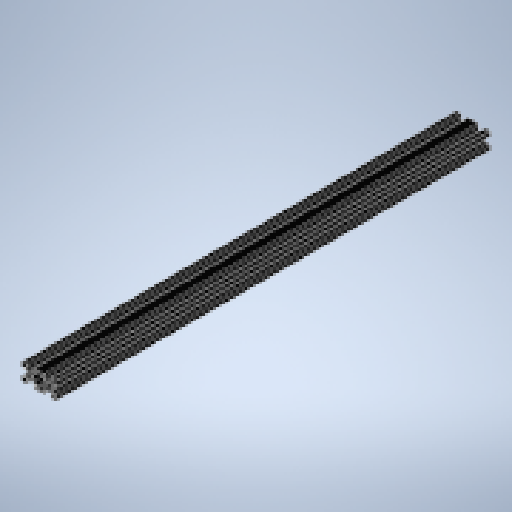
# Autodesk Inventor part: V-Slot_20x40_500
Saved by Autodesk Inventor 2025.1 (Build 291241020, 241B)
## iProperties
Created: 2017-01-26
Part Number: V-Slot_20x40_500
Material: Aluminum 6061
Document SubType Name: Modeling
Designer: leon-
Density: 2.7 g/cm^3
Appearance: Anodized - Black
Sending System: SolidWorks 2019
Last Author: ricardo
Last Saved: 2020-01-30
Author: leon-
Autodesk Inventor part; units mm, degrees
ref_plane "YZ Plane" through (0, 0, 0) normal (1, 0, 0) x (0, 1, 0)
ref_plane "XZ Plane" through (0, 0, 0) normal (0, 1, 0) x (-1, 0, 0)
ref_plane "Work Plane2" through (-5.2, 10, 100) normal (0, 0, 1) x (1, 0, 0)
sketch "Sketch1" plane through (-5.2, 10, 100) normal (0, 0, 1) x (1, 0, 0)
  line L0 (7.9, -18.2) -> (7.9, -16.2393) projected
  line L1 (2.5, -18.2) -> (7.9, -18.2) projected
  line L2 (2.5, -18.2) -> (2.5, -16.2393) projected
  line L3 (2.5, -16.2393) -> (-0.8, -12.9393) projected
  line L4 (-0.8, -7.0607) -> (-0.8, -12.9393) projected
  line L5 (2.5, -3.7607) -> (-0.8, -7.0607) projected
  line L6 (12.2, -18.2) -> (9.7, -18.2) projected
  line L7 (10.4, -20) -> (12.2, -18.2) projected
  line L8 (0, -20) -> (10.4, -20) projected
  line L9 (0, -20) -> (-1.8, -18.2) projected
  line L10 (-1.8, -18.2) -> (0.7, -18.2) projected
  line L11 (0.7, -18.2) -> (0.7, -16.5607) projected
  line L12 (0.7, -16.5607) -> (-1.8607, -14) projected
  line L13 (-1.8607, -14) -> (-4.5, -14) projected
  line L14 (-4.5, -14) -> (-4.8, -13.7) projected
  line L15 (-5.1, -14) -> (-4.8, -13.7) projected
  line L16 (-5.1, -14) -> (-7.7393, -14) projected
  line L17 (-10.3, -16.5607) -> (-7.7393, -14) projected
  line L18 (-10.3, -18.2) -> (-10.3, -16.5607) projected
  line L19 (-7.8, -18.2) -> (-10.3, -18.2) projected
  line L20 (-9.6, -20) -> (-7.8, -18.2) projected
  line L21 (-13.8, -20) -> (-9.6, -20) projected
  arc A0 (-14.8, -19) -> (-13.8, -20) centre (-13.8, -19) ccw projected
  line L22 (-14.8, -14.8) -> (-14.8, -19) projected
  line L23 (-14.8, -14.8) -> (-13, -13) projected
  line L24 (-13, -13) -> (-13, -15.5) projected
  line L25 (-13, -15.5) -> (-11.3607, -15.5) projected
  line L26 (-11.3607, -15.5) -> (-8.8, -12.9393) projected
  line L27 (-8.8, -12.9393) -> (-8.8, -10.3) projected
  line L28 (-8.8, -10.3) -> (-8.5, -10) projected
  line L29 (-8.8, -9.7) -> (-8.5, -10) projected
  line L30 (-8.8, -9.7) -> (-8.8, -7.0607) projected
  line L31 (-11.3607, -4.5) -> (-8.8, -7.0607) projected
  line L32 (-13, -4.5) -> (-11.3607, -4.5) projected
  line L33 (-13, -7) -> (-13, -4.5) projected
  line L34 (-14.8, -5.2) -> (-13, -7) projected
  line L35 (-14.8, -1) -> (-14.8, -5.2) projected
  arc A1 (-13.8, 0) -> (-14.8, -1) centre (-13.8, -1) ccw projected
  line L36 (-9.6, 0) -> (-13.8, 0) projected
  line L37 (-9.6, 0) -> (-7.8, -1.8) projected
  line L38 (-7.8, -1.8) -> (-10.3, -1.8) projected
  line L39 (-10.3, -1.8) -> (-10.3, -3.4393) projected
  line L40 (-10.3, -3.4393) -> (-7.7393, -6) projected
  line L41 (-7.7393, -6) -> (-5.1, -6) projected
  line L42 (-5.1, -6) -> (-4.8, -6.3) projected
  line L43 (-4.5, -6) -> (-4.8, -6.3) projected
  line L44 (-4.5, -6) -> (-1.8607, -6) projected
  line L45 (0.7, -3.4393) -> (-1.8607, -6) projected
  line L46 (0.7, -1.8) -> (0.7, -3.4393) projected
  line L47 (-1.8, -1.8) -> (0.7, -1.8) projected
  line L48 (0, 0) -> (-1.8, -1.8) projected
  line L49 (10.4, 0) -> (0, 0) projected
  line L50 (10.4, 0) -> (12.2, -1.8) projected
  line L51 (12.2, -1.8) -> (9.7, -1.8) projected
  line L52 (9.7, -1.8) -> (9.7, -3.4393) projected
  line L53 (9.7, -3.4393) -> (12.2607, -6) projected
  line L54 (14.9, -6) -> (12.2607, -6) projected
  line L55 (14.9, -6) -> (15.2, -6.3) projected
  line L56 (15.5, -6) -> (15.2, -6.3) projected
  line L57 (18.1393, -6) -> (15.5, -6) projected
  line L58 (20.7, -3.4393) -> (18.1393, -6) projected
  line L59 (20.7, -1.8) -> (20.7, -3.4393) projected
  line L60 (18.2, -1.8) -> (20.7, -1.8) projected
  line L61 (20, 0) -> (18.2, -1.8) projected
  line L62 (24.2, 0) -> (20, 0) projected
  arc A2 (25.2, -1) -> (24.2, 0) centre (24.2, -1) ccw projected
  line L63 (25.2, -5.2) -> (25.2, -1) projected
  line L64 (25.2, -5.2) -> (23.4, -7) projected
  line L65 (23.4, -7) -> (23.4, -4.5) projected
  line L66 (23.4, -4.5) -> (21.7607, -4.5) projected
  line L67 (21.7607, -4.5) -> (19.2, -7.0607) projected
  line L68 (19.2, -9.7) -> (19.2, -7.0607) projected
  line L69 (19.2, -9.7) -> (18.9, -10) projected
  line L70 (19.2, -10.3) -> (18.9, -10) projected
  line L71 (19.2, -12.9393) -> (19.2, -10.3) projected
  line L72 (21.7607, -15.5) -> (19.2, -12.9393) projected
  line L73 (23.4, -15.5) -> (21.7607, -15.5) projected
  line L74 (23.4, -13) -> (23.4, -15.5) projected
  line L75 (25.2, -14.8) -> (23.4, -13) projected
  line L76 (25.2, -19) -> (25.2, -14.8) projected
  arc A3 (24.2, -20) -> (25.2, -19) centre (24.2, -19) ccw projected
  line L77 (20, -20) -> (24.2, -20) projected
  line L78 (20, -20) -> (18.2, -18.2) projected
  line L79 (18.2, -18.2) -> (20.7, -18.2) projected
  line L80 (20.7, -18.2) -> (20.7, -16.5607) projected
  line L81 (20.7, -16.5607) -> (18.1393, -14) projected
  line L82 (15.5, -14) -> (18.1393, -14) projected
  line L83 (15.5, -14) -> (15.2, -13.7) projected
  line L84 (14.9, -14) -> (15.2, -13.7) projected
  line L85 (12.2607, -14) -> (14.9, -14) projected
  line L86 (9.7, -16.5607) -> (12.2607, -14) projected
  line L87 (9.7, -18.2) -> (9.7, -16.5607) projected
  circle A4 centre (15.2, -10) radius 2.1 projected
  circle A5 centre (-4.8, -10) radius 2.1 projected
  line L88 (7.9, -16.2393) -> (11.2, -12.9393) projected
  line L89 (11.2, -7.0607) -> (11.2, -12.9393) projected
  line L90 (7.9, -3.7607) -> (11.2, -7.0607) projected
  line L91 (7.9, -1.8) -> (7.9, -3.7607) projected
  line L92 (2.5, -1.8) -> (7.9, -1.8) projected
  line L93 (2.5, -1.8) -> (2.5, -3.7607) projected
  line L94 (2.5, -3.7607) -> (-0.8, -7.0607) projected
  line L95 (-0.8, -7.0607) -> (-0.8, -12.9393) projected
  line L96 (2.5, -16.2393) -> (-0.8, -12.9393) projected
  line L97 (2.5, -18.2) -> (2.5, -16.2393) projected
  line L98 (2.5, -18.2) -> (7.9, -18.2) projected
  line L99 (7.9, -18.2) -> (7.9, -16.2393) projected
  line L100 (0.7, -18.2) -> (0.7, -16.5607) projected
  line L101 (0.7, -16.5607) -> (-1.8607, -14) projected
  line L102 (-1.8, -18.2) -> (0.7, -18.2) projected
  line L103 (0, -20) -> (-1.8, -18.2) projected
  line L104 (-1.8607, -14) -> (-4.5, -14) projected
  line L105 (-4.5, -14) -> (-4.8, -13.7) projected
  line L106 (-5.1, -14) -> (-4.8, -13.7) projected
  circle A6 centre (-4.8, -10) radius 2.1 projected
  line L107 (-5.1, -14) -> (-7.7393, -14) projected
  line L108 (-8.8, -9.7) -> (-8.5, -10) projected
  line L109 (-8.8, -12.9393) -> (-8.8, -10.3) projected
  line L110 (-8.8, -9.7) -> (-8.8, -7.0607) projected
  line L111 (-10.3, -16.5607) -> (-7.7393, -14) projected
  line L112 (-10.3, -18.2) -> (-10.3, -16.5607) projected
  line L113 (-13, -15.5) -> (-11.3607, -15.5) projected
  line L114 (-13, -13) -> (-13, -15.5) projected
  line L115 (-14.8, -14.8) -> (-14.8, -19) projected
  line L116 (-11.3607, -4.5) -> (-8.8, -7.0607) projected
  line L117 (-13, -7) -> (-13, -4.5) projected
  line L118 (0.7, -3.4393) -> (-1.8607, -6) projected
  line L119 (2.5, -1.8) -> (2.5, -3.7607) projected
  line L120 (2.5, -1.8) -> (7.9, -1.8) projected
  line L121 (7.9, -1.8) -> (7.9, -3.7607) projected
  line L122 (9.7, -18.2) -> (9.7, -16.5607) projected
  line L123 (7.9, -3.7607) -> (11.2, -7.0607) projected
  line L124 (7.9, -16.2393) -> (11.2, -12.9393) projected
  line L125 (11.2, -7.0607) -> (11.2, -12.9393) projected
  line L126 (9.7, -16.5607) -> (12.2607, -14) projected
  line L127 (12.2607, -14) -> (14.9, -14) projected
  line L128 (14.9, -14) -> (15.2, -13.7) projected
  circle A7 centre (15.2, -10) radius 2.1 projected
  line L129 (15.5, -14) -> (15.2, -13.7) projected
  line L130 (-13, -4.5) -> (-11.3607, -4.5) projected
  line L131 (15.5, -14) -> (18.1393, -14) projected
  line L132 (19.2, -12.9393) -> (19.2, -10.3) projected
  line L133 (20, -20) -> (18.2, -18.2) projected
  line L134 (20.7, -16.5607) -> (18.1393, -14) projected
  line L135 (18.2, -18.2) -> (20.7, -18.2) projected
  line L136 (20.7, -18.2) -> (20.7, -16.5607) projected
  line L137 (21.7607, -15.5) -> (19.2, -12.9393) projected
  line L138 (23.4, -15.5) -> (21.7607, -15.5) projected
  arc A8 (24.2, -20) -> (25.2, -19) centre (24.2, -19) ccw projected
  line L139 (25.2, -19) -> (25.2, -14.8) projected
  line L140 (25.2, -14.8) -> (23.4, -13) projected
  line L141 (23.4, -13) -> (23.4, -15.5) projected
  line L142 (-7.8, -18.2) -> (-10.3, -18.2) projected
  arc A9 (-14.8, -19) -> (-13.8, -20) centre (-13.8, -19) ccw projected
  line L143 (-9.6, -20) -> (-7.8, -18.2) projected
  line L144 (-14.8, -14.8) -> (-13, -13) projected
  line L145 (-11.3607, -15.5) -> (-8.8, -12.9393) projected
  line L146 (-8.8, -10.3) -> (-8.5, -10) projected
  line L147 (19.2, -10.3) -> (18.9, -10) projected
  line L148 (19.2, -9.7) -> (18.9, -10) projected
  line L149 (19.2, -9.7) -> (19.2, -7.0607) projected
  line L150 (21.7607, -4.5) -> (19.2, -7.0607) projected
  line L151 (23.4, -4.5) -> (21.7607, -4.5) projected
  line L152 (23.4, -7) -> (23.4, -4.5) projected
  line L153 (25.2, -5.2) -> (23.4, -7) projected
  arc A10 (25.2, -1) -> (24.2, 0) centre (24.2, -1) ccw projected
  line L154 (20, 0) -> (18.2, -1.8) projected
  line L155 (18.2, -1.8) -> (20.7, -1.8) projected
  line L156 (15.5, -6) -> (15.2, -6.3) projected
  line L157 (18.1393, -6) -> (15.5, -6) projected
  line L158 (20.7, -3.4393) -> (18.1393, -6) projected
  line L159 (20.7, -1.8) -> (20.7, -3.4393) projected
  line L160 (0.7, -1.8) -> (0.7, -3.4393) projected
  line L161 (9.7, -3.4393) -> (12.2607, -6) projected
  line L162 (14.9, -6) -> (12.2607, -6) projected
  line L163 (14.9, -6) -> (15.2, -6.3) projected
  line L164 (9.7, -1.8) -> (9.7, -3.4393) projected
  line L165 (-1.8, -1.8) -> (0.7, -1.8) projected
  line L166 (12.2, -1.8) -> (9.7, -1.8) projected
  line L167 (10.4, 0) -> (12.2, -1.8) projected
  line L168 (0, 0) -> (-1.8, -1.8) projected
  line L169 (10.4, 0) -> (0, 0) projected
  line L170 (-14.8, -5.2) -> (-13, -7) projected
  line L171 (0, -20) -> (10.4, -20) projected
  line L172 (12.2, -18.2) -> (9.7, -18.2) projected
  line L173 (10.4, -20) -> (12.2, -18.2) projected
  line L174 (-7.8, -1.8) -> (-10.3, -1.8) projected
  line L175 (-9.6, 0) -> (-7.8, -1.8) projected
  line L176 (-9.6, 0) -> (-13.8, 0) projected
  arc A11 (-13.8, 0) -> (-14.8, -1) centre (-13.8, -1) ccw projected
  line L177 (-7.7393, -6) -> (-5.1, -6) projected
  line L178 (-10.3, -3.4393) -> (-7.7393, -6) projected
  line L179 (-10.3, -1.8) -> (-10.3, -3.4393) projected
  line L180 (-5.1, -6) -> (-4.8, -6.3) projected
  line L181 (-4.5, -6) -> (-4.8, -6.3) projected
  line L182 (-4.5, -6) -> (-1.8607, -6) projected
  line L183 (21.7607, -15.5) -> (19.2, -12.9393) projected
  line L184 (25.2, -14.8) -> (23.4, -13) projected
  arc A12 (24.2, -20) -> (25.2, -19) centre (24.2, -19) ccw projected
  line L185 (23.4, -7) -> (23.4, -4.5) projected
  line L186 (23.4, -4.5) -> (21.7607, -4.5) projected
  line L187 (21.7607, -4.5) -> (19.2, -7.0607) projected
  line L188 (19.2, -9.7) -> (19.2, -7.0607) projected
  line L189 (19.2, -9.7) -> (18.9, -10) projected
  line L190 (19.2, -10.3) -> (18.9, -10) projected
  line L191 (19.2, -12.9393) -> (19.2, -10.3) projected
  line L192 (25.2, -19) -> (25.2, -14.8) projected
  line L193 (23.4, -13) -> (23.4, -15.5) projected
  line L194 (23.4, -15.5) -> (21.7607, -15.5) projected
  line L195 (20.7, -18.2) -> (20.7, -16.5607) projected
  line L196 (18.2, -18.2) -> (20.7, -18.2) projected
  line L197 (20, -20) -> (18.2, -18.2) projected
  line L198 (2.5, -3.7607) -> (-0.8, -7.0607) projected
  line L199 (2.5, -3.7607) -> (-0.8, -7.0607) projected
  line L200 (2.5, -3.7607) -> (-0.8, -7.0607) projected
  line L201 (7.9, -3.7607) -> (11.2, -7.0607) projected
  line L202 (7.9, -3.7607) -> (11.2, -7.0607) projected
  line L203 (7.9, -3.7607) -> (11.2, -7.0607) projected
  line L204 (0.7, -3.4393) -> (-1.8607, -6) projected
  line L205 (0.7, -3.4393) -> (-1.8607, -6) projected
  line L206 (2.5, -1.8) -> (2.5, -3.7607) projected
  line L207 (2.5, -1.8) -> (2.5, -3.7607) projected
  line L208 (7.9, -1.8) -> (7.9, -3.7607) projected
  line L209 (7.9, -1.8) -> (7.9, -3.7607) projected
  line L210 (0.7, -1.8) -> (0.7, -3.4393) projected
  line L211 (0.7, -1.8) -> (0.7, -3.4393) projected
  line L212 (2.5, -1.8) -> (7.9, -1.8) projected
  line L213 (10.4, 0) -> (0, 0) projected
  line L214 (10.4, 0) -> (0, 0) projected
  line L215 (10.4, 0) -> (12.2, -1.8) projected
  line L216 (10.4, 0) -> (12.2, -1.8) projected
  line L217 (2.5, -1.8) -> (7.9, -1.8) projected
  line L218 (2.5, -1.8) -> (7.9, -1.8) projected
  line L219 (11.2, -7.0607) -> (11.2, -12.9393) projected
  line L220 (-0.8, -7.0607) -> (-0.8, -12.9393) projected
  line L221 (-0.8, -7.0607) -> (-0.8, -12.9393) projected
  line L222 (-0.8, -7.0607) -> (-0.8, -12.9393) projected
  line L223 (7.9, -16.2393) -> (11.2, -12.9393) projected
  line L224 (7.9, -16.2393) -> (11.2, -12.9393) projected
  line L225 (7.9, -16.2393) -> (11.2, -12.9393) projected
  line L226 (2.5, -18.2) -> (7.9, -18.2) projected
  line L227 (2.5, -18.2) -> (7.9, -18.2) projected
  line L228 (7.9, -18.2) -> (7.9, -16.2393) projected
  line L229 (7.9, -18.2) -> (7.9, -16.2393) projected
  line L230 (7.9, -18.2) -> (7.9, -16.2393) projected
  line L231 (2.5, -18.2) -> (2.5, -16.2393) projected
  line L232 (2.5, -18.2) -> (2.5, -16.2393) projected
  line L233 (2.5, -18.2) -> (2.5, -16.2393) projected
  line L234 (2.5, -16.2393) -> (-0.8, -12.9393) projected
  line L235 (2.5, -16.2393) -> (-0.8, -12.9393) projected
  line L236 (2.5, -16.2393) -> (-0.8, -12.9393) projected
  line L237 (0.7, -16.5607) -> (-1.8607, -14) projected
  line L238 (0.7, -16.5607) -> (-1.8607, -14) projected
  line L239 (0, 0) -> (-1.8, -1.8) projected
  line L240 (0, 0) -> (-1.8, -1.8) projected
  line L241 (-1.8, -1.8) -> (0.7, -1.8) projected
  line L242 (-1.8, -1.8) -> (0.7, -1.8) projected
  line L243 (23.4, -15.5) -> (21.7607, -15.5) projected
  line L244 (23.4, -15.5) -> (21.7607, -15.5) projected
  line L245 (23.4, -13) -> (23.4, -15.5) projected
  line L246 (23.4, -13) -> (23.4, -15.5) projected
  line L247 (25.2, -14.8) -> (23.4, -13) projected
  line L248 (25.2, -14.8) -> (23.4, -13) projected
  line L249 (21.7607, -15.5) -> (19.2, -12.9393) projected
  line L250 (21.7607, -15.5) -> (19.2, -12.9393) projected
  line L251 (18.2, -18.2) -> (20.7, -18.2) projected
  line L252 (18.2, -18.2) -> (20.7, -18.2) projected
  line L253 (20, -20) -> (18.2, -18.2) projected
  line L254 (20, -20) -> (18.2, -18.2) projected
  line L255 (20, -20) -> (24.2, -20) projected
  line L256 (20, -20) -> (24.2, -20) projected
  line L257 (20.7, -18.2) -> (20.7, -16.5607) projected
  line L258 (20.7, -18.2) -> (20.7, -16.5607) projected
  line L259 (24.2, 0) -> (20, 0) projected
  line L260 (24.2, 0) -> (20, 0) projected
  line L261 (25.2, -5.2) -> (25.2, -1) projected
  line L262 (9.7, -18.2) -> (9.7, -16.5607) projected
  line L263 (9.7, -18.2) -> (9.7, -16.5607) projected
  line L264 (10.4, -20) -> (12.2, -18.2) projected
  line L265 (10.4, -20) -> (12.2, -18.2) projected
  line L266 (12.2, -18.2) -> (9.7, -18.2) projected
  line L267 (12.2, -18.2) -> (9.7, -18.2) projected
  line L268 (9.7, -16.5607) -> (12.2607, -14) projected
  line L269 (9.7, -16.5607) -> (12.2607, -14) projected
  line L270 (9.7, -16.5607) -> (12.2607, -14) projected
  line L271 (12.2607, -14) -> (14.9, -14) projected
  line L272 (14.9, -14) -> (15.2, -13.7) projected
  line L273 (15.5, -14) -> (15.2, -13.7) projected
  line L274 (15.5, -14) -> (18.1393, -14) projected
  line L275 (20.7, -16.5607) -> (18.1393, -14) projected
  line L276 (11.2, -7.0607) -> (11.2, -12.9393) projected
  line L277 (11.2, -7.0607) -> (11.2, -12.9393) projected
  line L278 (12.2607, -14) -> (14.9, -14) projected
  line L279 (12.2607, -14) -> (14.9, -14) projected
  line L280 (14.9, -14) -> (15.2, -13.7) projected
  line L281 (14.9, -14) -> (15.2, -13.7) projected
  line L282 (15.5, -14) -> (15.2, -13.7) projected
  line L283 (15.5, -14) -> (15.2, -13.7) projected
  line L284 (20, 0) -> (18.2, -1.8) projected
  line L285 (20, 0) -> (18.2, -1.8) projected
  line L286 (19.2, -9.7) -> (19.2, -7.0607) projected
  line L287 (19.2, -9.7) -> (19.2, -7.0607) projected
  line L288 (19.2, -9.7) -> (18.9, -10) projected
  line L289 (19.2, -9.7) -> (18.9, -10) projected
  line L290 (19.2, -10.3) -> (18.9, -10) projected
  line L291 (19.2, -10.3) -> (18.9, -10) projected
  line L292 (21.7607, -4.5) -> (19.2, -7.0607) projected
  line L293 (21.7607, -4.5) -> (19.2, -7.0607) projected
  line L294 (23.4, -7) -> (23.4, -4.5) projected
  line L295 (23.4, -7) -> (23.4, -4.5) projected
  line L296 (23.4, -4.5) -> (21.7607, -4.5) projected
  line L297 (23.4, -4.5) -> (21.7607, -4.5) projected
  line L298 (15.5, -14) -> (18.1393, -14) projected
  line L299 (15.5, -14) -> (18.1393, -14) projected
  line L300 (19.2, -12.9393) -> (19.2, -10.3) projected
  line L301 (19.2, -12.9393) -> (19.2, -10.3) projected
  line L302 (20.7, -16.5607) -> (18.1393, -14) projected
  line L303 (20.7, -16.5607) -> (18.1393, -14) projected
  circle A13 centre (15.2, -10) radius 2.1 projected
  circle A14 centre (15.2, -10) radius 2.1 projected
  line L304 (9.7, -1.8) -> (9.7, -3.4393) projected
  line L305 (9.7, -1.8) -> (9.7, -3.4393) projected
  line L306 (9.7, -3.4393) -> (12.2607, -6) projected
  line L307 (9.7, -3.4393) -> (12.2607, -6) projected
  line L308 (14.9, -6) -> (12.2607, -6) projected
  line L309 (14.9, -6) -> (12.2607, -6) projected
  line L310 (14.9, -6) -> (15.2, -6.3) projected
  line L311 (14.9, -6) -> (15.2, -6.3) projected
  line L312 (15.5, -6) -> (15.2, -6.3) projected
  line L313 (15.5, -6) -> (15.2, -6.3) projected
  line L314 (18.1393, -6) -> (15.5, -6) projected
  line L315 (18.1393, -6) -> (15.5, -6) projected
  line L316 (20.7, -3.4393) -> (18.1393, -6) projected
  line L317 (20.7, -3.4393) -> (18.1393, -6) projected
  line L318 (20.7, -1.8) -> (20.7, -3.4393) projected
  line L319 (20.7, -1.8) -> (20.7, -3.4393) projected
  line L320 (18.2, -1.8) -> (20.7, -1.8) projected
  line L321 (18.2, -1.8) -> (20.7, -1.8) projected
  line L322 (12.2, -1.8) -> (9.7, -1.8) projected
  line L323 (12.2, -1.8) -> (9.7, -1.8) projected
  line L324 (7.9, -1.8) -> (7.9, -3.7607) projected
  line L325 (0.7, -18.2) -> (0.7, -16.5607) projected
  line L326 (0.7, -18.2) -> (0.7, -16.5607) projected
  line L327 (-1.8, -18.2) -> (0.7, -18.2) projected
  line L328 (-1.8, -18.2) -> (0.7, -18.2) projected
  line L329 (0, -20) -> (10.4, -20) projected
  line L330 (0, -20) -> (10.4, -20) projected
  line L331 (0, -20) -> (-1.8, -18.2) projected
  line L332 (0, -20) -> (-1.8, -18.2) projected
  line L333 (-13.8, -20) -> (-9.6, -20) projected
  arc A15 (-14.8, -19) -> (-13.8, -20) centre (-13.8, -19) ccw projected
  line L334 (25.2, -5.2) -> (23.4, -7) projected
  line L335 (25.2, -5.2) -> (23.4, -7) projected
  line L336 (24.2, 0) -> (20, 0) projected
  line L337 (24.2, 0) -> (20, 0) projected
  arc A16 (25.2, -1) -> (24.2, 0) centre (24.2, -1) ccw projected
  arc A17 (25.2, -1) -> (24.2, 0) centre (24.2, -1) ccw projected
  line L338 (25.2, -5.2) -> (25.2, -1) projected
  line L339 (25.2, -5.2) -> (25.2, -1) projected
  line L340 (25.2, -19) -> (25.2, -14.8) projected
  line L341 (25.2, -19) -> (25.2, -14.8) projected
  arc A18 (24.2, -20) -> (25.2, -19) centre (24.2, -19) ccw projected
  arc A19 (24.2, -20) -> (25.2, -19) centre (24.2, -19) ccw projected
  line L342 (20, -20) -> (24.2, -20) projected
  line L343 (20, -20) -> (24.2, -20) projected
  line L344 (2.5, -1.8) -> (2.5, -3.7607) projected
  line L345 (-4.5, -14) -> (-4.8, -13.7) projected
  line L346 (-5.1, -14) -> (-7.7393, -14) projected
  line L347 (-5.1, -14) -> (-4.8, -13.7) projected
  line L348 (-10.3, -16.5607) -> (-7.7393, -14) projected
  line L349 (-7.8, -18.2) -> (-10.3, -18.2) projected
  line L350 (0.7, -16.5607) -> (-1.8607, -14) projected
  line L351 (9.7, -1.8) -> (9.7, -3.4393) projected
  line L352 (9.7, -3.4393) -> (12.2607, -6) projected
  line L353 (2.5, -18.2) -> (7.9, -18.2) projected
  line L354 (20, 0) -> (18.2, -1.8) projected
  arc A20 (25.2, -1) -> (24.2, 0) centre (24.2, -1) ccw projected
  line L355 (12.2, -1.8) -> (9.7, -1.8) projected
  line L356 (25.2, -5.2) -> (23.4, -7) projected
  line L357 (25.2, -5.2) -> (25.2, -1) projected
  line L358 (10.4, 0) -> (12.2, -1.8) projected
  line L359 (10.4, 0) -> (0, 0) projected
  line L360 (10.4, -20) -> (12.2, -18.2) projected
  line L361 (12.2, -18.2) -> (9.7, -18.2) projected
  line L362 (9.7, -18.2) -> (9.7, -16.5607) projected
  line L363 (9.7, -16.5607) -> (12.2607, -14) projected
  line L364 (12.2607, -14) -> (14.9, -14) projected
  line L365 (14.9, -14) -> (15.2, -13.7) projected
  line L366 (15.5, -14) -> (15.2, -13.7) projected
  line L367 (15.5, -14) -> (18.1393, -14) projected
  line L368 (20.7, -16.5607) -> (18.1393, -14) projected
  line L369 (20.7, -18.2) -> (20.7, -16.5607) projected
  line L370 (18.2, -18.2) -> (20.7, -18.2) projected
  line L371 (20, -20) -> (18.2, -18.2) projected
  line L372 (20, -20) -> (24.2, -20) projected
  arc A21 (24.2, -20) -> (25.2, -19) centre (24.2, -19) ccw projected
  line L373 (25.2, -19) -> (25.2, -14.8) projected
  line L374 (25.2, -14.8) -> (23.4, -13) projected
  line L375 (23.4, -13) -> (23.4, -15.5) projected
  line L376 (23.4, -15.5) -> (21.7607, -15.5) projected
  line L377 (21.7607, -15.5) -> (19.2, -12.9393) projected
  line L378 (19.2, -12.9393) -> (19.2, -10.3) projected
  line L379 (19.2, -10.3) -> (18.9, -10) projected
  line L380 (19.2, -9.7) -> (18.9, -10) projected
  line L381 (19.2, -9.7) -> (19.2, -7.0607) projected
  line L382 (21.7607, -4.5) -> (19.2, -7.0607) projected
  line L383 (23.4, -4.5) -> (21.7607, -4.5) projected
  line L384 (23.4, -7) -> (23.4, -4.5) projected
  line L385 (25.2, -5.2) -> (23.4, -7) projected
  line L386 (25.2, -5.2) -> (25.2, -1) projected
  arc A22 (25.2, -1) -> (24.2, 0) centre (24.2, -1) ccw projected
  line L387 (24.2, 0) -> (20, 0) projected
  line L388 (20, 0) -> (18.2, -1.8) projected
  line L389 (18.2, -1.8) -> (20.7, -1.8) projected
  line L390 (20.7, -1.8) -> (20.7, -3.4393) projected
  line L391 (20.7, -3.4393) -> (18.1393, -6) projected
  line L392 (18.1393, -6) -> (15.5, -6) projected
  line L393 (15.5, -6) -> (15.2, -6.3) projected
  line L394 (14.9, -6) -> (15.2, -6.3) projected
  line L395 (14.9, -6) -> (12.2607, -6) projected
  line L396 (9.7, -3.4393) -> (12.2607, -6) projected
  line L397 (9.7, -1.8) -> (9.7, -3.4393) projected
  line L398 (12.2, -1.8) -> (9.7, -1.8) projected
  line L399 (10.4, 0) -> (12.2, -1.8) projected
  line L400 (10.4, 0) -> (0, 0) projected
  line L401 (0, 0) -> (-1.8, -1.8) projected
  line L402 (-1.8, -1.8) -> (0.7, -1.8) projected
  line L403 (0.7, -1.8) -> (0.7, -3.4393) projected
  line L404 (0.7, -3.4393) -> (-1.8607, -6) projected
  line L405 (-4.5, -6) -> (-1.8607, -6) projected
  line L406 (-4.5, -6) -> (-4.8, -6.3) projected
  line L407 (-5.1, -6) -> (-4.8, -6.3) projected
  line L408 (-7.7393, -6) -> (-5.1, -6) projected
  line L409 (-10.3, -3.4393) -> (-7.7393, -6) projected
  line L410 (-10.3, -1.8) -> (-10.3, -3.4393) projected
  line L411 (-7.8, -1.8) -> (-10.3, -1.8) projected
  line L412 (-9.6, 0) -> (-7.8, -1.8) projected
  line L413 (-9.6, 0) -> (-13.8, 0) projected
  arc A23 (-13.8, 0) -> (-14.8, -1) centre (-13.8, -1) ccw projected
  line L414 (-14.8, -1) -> (-14.8, -5.2) projected
  line L415 (-14.8, -5.2) -> (-13, -7) projected
  line L416 (-13, -7) -> (-13, -4.5) projected
  line L417 (-13, -4.5) -> (-11.3607, -4.5) projected
  line L418 (-11.3607, -4.5) -> (-8.8, -7.0607) projected
  line L419 (-8.8, -9.7) -> (-8.8, -7.0607) projected
  line L420 (-8.8, -9.7) -> (-8.5, -10) projected
  line L421 (-8.8, -10.3) -> (-8.5, -10) projected
  line L422 (-8.8, -12.9393) -> (-8.8, -10.3) projected
  line L423 (-11.3607, -15.5) -> (-8.8, -12.9393) projected
  line L424 (-13, -15.5) -> (-11.3607, -15.5) projected
  line L425 (-13, -13) -> (-13, -15.5) projected
  line L426 (-14.8, -14.8) -> (-13, -13) projected
  line L427 (-14.8, -14.8) -> (-14.8, -19) projected
  arc A24 (-14.8, -19) -> (-13.8, -20) centre (-13.8, -19) ccw projected
  line L428 (-13.8, -20) -> (-9.6, -20) projected
  line L429 (-9.6, -20) -> (-7.8, -18.2) projected
  line L430 (-7.8, -18.2) -> (-10.3, -18.2) projected
  line L431 (-10.3, -18.2) -> (-10.3, -16.5607) projected
  line L432 (-10.3, -16.5607) -> (-7.7393, -14) projected
  line L433 (-5.1, -14) -> (-7.7393, -14) projected
  line L434 (-5.1, -14) -> (-4.8, -13.7) projected
  line L435 (-4.5, -14) -> (-4.8, -13.7) projected
  line L436 (-1.8607, -14) -> (-4.5, -14) projected
  line L437 (0.7, -16.5607) -> (-1.8607, -14) projected
  line L438 (0.7, -18.2) -> (0.7, -16.5607) projected
  line L439 (-1.8, -18.2) -> (0.7, -18.2) projected
  line L440 (0, -20) -> (-1.8, -18.2) projected
  line L441 (0, -20) -> (10.4, -20) projected
  circle A25 centre (15.2, -10) radius 2.1 projected
  circle A26 centre (-4.8, -10) radius 2.1 projected
  line L442 (11.2, -7.0607) -> (11.2, -12.9393) projected
  line L443 (7.9, -16.2393) -> (11.2, -12.9393) projected
  line L444 (7.9, -18.2) -> (7.9, -16.2393) projected
  line L445 (2.5, -18.2) -> (7.9, -18.2) projected
  line L446 (2.5, -18.2) -> (2.5, -16.2393) projected
  line L447 (2.5, -16.2393) -> (-0.8, -12.9393) projected
  line L448 (-0.8, -7.0607) -> (-0.8, -12.9393) projected
  line L449 (2.5, -3.7607) -> (-0.8, -7.0607) projected
  line L450 (2.5, -1.8) -> (2.5, -3.7607) projected
  line L451 (2.5, -1.8) -> (7.9, -1.8) projected
  line L452 (7.9, -1.8) -> (7.9, -3.7607) projected
  line L453 (7.9, -3.7607) -> (11.2, -7.0607) projected
  line L454 (0.7, -1.8) -> (0.7, -3.4393) projected
  line L455 (-1.8, -1.8) -> (0.7, -1.8) projected
  line L456 (0.7, -3.4393) -> (-1.8607, -6) projected
  line L457 (0, 0) -> (-1.8, -1.8) projected
  line L458 (-4.5, -6) -> (-1.8607, -6) projected
  line L459 (-4.5, -6) -> (-4.8, -6.3) projected
  line L460 (-5.1, -6) -> (-4.8, -6.3) projected
  line L461 (-7.7393, -6) -> (-5.1, -6) projected
  line L462 (-8.8, -9.7) -> (-8.8, -7.0607) projected
  line L463 (-8.8, -9.7) -> (-8.5, -10) projected
  line L464 (-9.6, 0) -> (-7.8, -1.8) projected
  line L465 (-8.8, -10.3) -> (-8.5, -10) projected
  line L466 (-10.3, -3.4393) -> (-7.7393, -6) projected
  line L467 (-7.8, -1.8) -> (-10.3, -1.8) projected
  line L468 (-10.3, -1.8) -> (-10.3, -3.4393) projected
  line L469 (-8.8, -12.9393) -> (-8.8, -10.3) projected
  line L470 (-11.3607, -4.5) -> (-8.8, -7.0607) projected
  line L471 (-9.6, 0) -> (-13.8, 0) projected
  arc A27 (-13.8, 0) -> (-14.8, -1) centre (-13.8, -1) ccw projected
  line L472 (-13, -4.5) -> (-11.3607, -4.5) projected
  line L473 (-11.3607, -15.5) -> (-8.8, -12.9393) projected
  line L474 (-14.8, -5.2) -> (-13, -7) projected
  line L475 (-13, -15.5) -> (-11.3607, -15.5) projected
  line L476 (-13, -13) -> (-13, -15.5) projected
  line L477 (-14.8, -14.8) -> (-13, -13) projected
  line L478 (-14.8, -14.8) -> (-14.8, -19) projected
  line L479 (-13, -7) -> (-13, -4.5) projected
  line L480 (20.7, -1.8) -> (20.7, -3.4393) projected
  line L481 (-10.3, -18.2) -> (-10.3, -16.5607) projected
  circle A28 centre (-4.8, -10) radius 2.1 projected
  line L482 (-1.8607, -14) -> (-4.5, -14) projected
  line L483 (-1.8, -18.2) -> (0.7, -18.2) projected
  line L484 (0, -20) -> (-1.8, -18.2) projected
  line L485 (0, -20) -> (10.4, -20) projected
  line L486 (0.7, -18.2) -> (0.7, -16.5607) projected
  line L487 (18.2, -1.8) -> (20.7, -1.8) projected
  line L488 (20.7, -3.4393) -> (18.1393, -6) projected
  circle A29 centre (15.2, -10) radius 2.1 projected
  line L489 (14.9, -6) -> (12.2607, -6) projected
  line L490 (18.1393, -6) -> (15.5, -6) projected
  line L491 (14.9, -6) -> (15.2, -6.3) projected
  line L492 (15.5, -6) -> (15.2, -6.3) projected
  line L493 (9.7, -18.2) -> (9.7, -16.5607) projected
  line L494 (10.4, -20) -> (12.2, -18.2) projected
  line L495 (-9.6, -20) -> (-7.8, -18.2) projected
  line L496 (12.2, -18.2) -> (9.7, -18.2) projected
  line L497 (-4.5, -6) -> (-1.8607, -6) projected
  line L498 (-4.5, -6) -> (-1.8607, -6) projected
  line L499 (-4.5, -6) -> (-4.8, -6.3) projected
  line L500 (-4.5, -6) -> (-4.8, -6.3) projected
  line L501 (-4.5, -14) -> (-4.8, -13.7) projected
  line L502 (-4.5, -14) -> (-4.8, -13.7) projected
  line L503 (-5.1, -6) -> (-4.8, -6.3) projected
  line L504 (-5.1, -6) -> (-4.8, -6.3) projected
  circle A30 centre (-4.8, -10) radius 2.1 projected
  circle A31 centre (-4.8, -10) radius 2.1 projected
  line L505 (-7.7393, -6) -> (-5.1, -6) projected
  line L506 (-7.7393, -6) -> (-5.1, -6) projected
  line L507 (-8.8, -9.7) -> (-8.5, -10) projected
  line L508 (-8.8, -9.7) -> (-8.5, -10) projected
  line L509 (-8.8, -10.3) -> (-8.5, -10) projected
  line L510 (-8.8, -10.3) -> (-8.5, -10) projected
  line L511 (-1.8607, -14) -> (-4.5, -14) projected
  line L512 (-1.8607, -14) -> (-4.5, -14) projected
  line L513 (-5.1, -14) -> (-7.7393, -14) projected
  line L514 (-5.1, -14) -> (-7.7393, -14) projected
  line L515 (-10.3, -16.5607) -> (-7.7393, -14) projected
  line L516 (-10.3, -16.5607) -> (-7.7393, -14) projected
  line L517 (-7.8, -18.2) -> (-10.3, -18.2) projected
  line L518 (-7.8, -18.2) -> (-10.3, -18.2) projected
  line L519 (-10.3, -18.2) -> (-10.3, -16.5607) projected
  line L520 (-10.3, -18.2) -> (-10.3, -16.5607) projected
  line L521 (-9.6, -20) -> (-7.8, -18.2) projected
  line L522 (-9.6, -20) -> (-7.8, -18.2) projected
  line L523 (-5.1, -14) -> (-4.8, -13.7) projected
  line L524 (-5.1, -14) -> (-4.8, -13.7) projected
  line L525 (-9.6, 0) -> (-7.8, -1.8) projected
  line L526 (-9.6, 0) -> (-7.8, -1.8) projected
  line L527 (-11.3607, -4.5) -> (-8.8, -7.0607) projected
  line L528 (-11.3607, -4.5) -> (-8.8, -7.0607) projected
  line L529 (-8.8, -12.9393) -> (-8.8, -10.3) projected
  line L530 (-8.8, -12.9393) -> (-8.8, -10.3) projected
  line L531 (-11.3607, -15.5) -> (-8.8, -12.9393) projected
  line L532 (-11.3607, -15.5) -> (-8.8, -12.9393) projected
  line L533 (-8.8, -9.7) -> (-8.8, -7.0607) projected
  line L534 (-8.8, -9.7) -> (-8.8, -7.0607) projected
  line L535 (-13.8, -20) -> (-9.6, -20) projected
  line L536 (-13.8, -20) -> (-9.6, -20) projected
  line L537 (-13.8, -20) -> (-9.6, -20) projected
  line L538 (-13, -13) -> (-13, -15.5) projected
  line L539 (-13, -13) -> (-13, -15.5) projected
  arc A32 (-14.8, -19) -> (-13.8, -20) centre (-13.8, -19) ccw projected
  arc A33 (-14.8, -19) -> (-13.8, -20) centre (-13.8, -19) ccw projected
  line L540 (-14.8, -14.8) -> (-14.8, -19) projected
  line L541 (-14.8, -14.8) -> (-14.8, -19) projected
  line L542 (-14.8, -14.8) -> (-13, -13) projected
  line L543 (-14.8, -14.8) -> (-13, -13) projected
  line L544 (-13, -15.5) -> (-11.3607, -15.5) projected
  line L545 (-13, -15.5) -> (-11.3607, -15.5) projected
  line L546 (-7.8, -1.8) -> (-10.3, -1.8) projected
  line L547 (-7.8, -1.8) -> (-10.3, -1.8) projected
  line L548 (-10.3, -1.8) -> (-10.3, -3.4393) projected
  line L549 (-10.3, -1.8) -> (-10.3, -3.4393) projected
  line L550 (-13, -7) -> (-13, -4.5) projected
  line L551 (-13, -7) -> (-13, -4.5) projected
  line L552 (-13, -4.5) -> (-11.3607, -4.5) projected
  line L553 (-13, -4.5) -> (-11.3607, -4.5) projected
  line L554 (-10.3, -3.4393) -> (-7.7393, -6) projected
  line L555 (-10.3, -3.4393) -> (-7.7393, -6) projected
  line L556 (-14.8, -5.2) -> (-13, -7) projected
  line L557 (-14.8, -5.2) -> (-13, -7) projected
  line L558 (-14.8, -1) -> (-14.8, -5.2) projected
  line L559 (-14.8, -1) -> (-14.8, -5.2) projected
  line L560 (-14.8, -1) -> (-14.8, -5.2) projected
  arc A34 (-13.8, 0) -> (-14.8, -1) centre (-13.8, -1) ccw projected
  arc A35 (-13.8, 0) -> (-14.8, -1) centre (-13.8, -1) ccw projected
  line L561 (-9.6, 0) -> (-13.8, 0) projected
  line L562 (-9.6, 0) -> (-13.8, 0) projected
  line L563 (-14.8, -1) -> (-14.8, -5.2) projected
  point P0 (5.2, -10)
  constraints: 32 other
extrude "Extrusion1" add sketch "Sketch1" along normal blind 500
body "Solid1"
